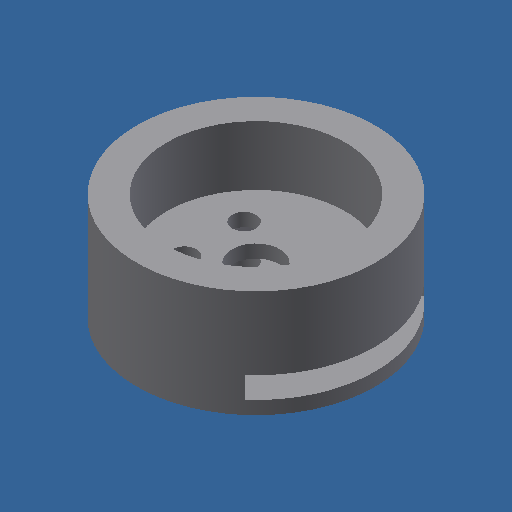
# Autodesk Inventor part: Acople_sensor_hall
Saved by Autodesk Inventor 2025 (Build 290162000, 162)
## iProperties
Created: 2025-09-16
Part Number: Acople_sensor_hall
Material: Generic
Document SubType Name: Modeling
Designer: HP
Density: 1 g/cm^3
Appearance: Default
Author: HP
Autodesk Inventor part; units mm, degrees
ref_plane "XZ Plane" through (0, 0, 0) normal (0, 1, 0) x (-1, 0, 0)
ref_plane "XY Plane" through (0, 0, 0) normal (0, 0, 1) x (1, 0, 0)
sketch "Boceto1" plane through (0, 0, 0) normal (0, 1, 0) x (-1, 0, 0)
  circle A0 centre (0, 0) radius 10
  circle A1 centre (0, 0) radius 7.5
  dimension "d0" = 20
  dimension "d1" = 15
  constraints: 2 centre point, 2 coincident
  measures "d0" diameter of A0
  measures "d1" diameter of A1
extrude "Extrusión1" add sketch "Boceto1" along normal blind 5
sketch "Boceto2" plane through (0, 0, 0) normal (0, -1, 0) x (1, 0, 0)
  circle A0 centre (0, 0) radius 10 projected
extrude "Extrusión2" add sketch "Boceto2" along normal blind 4
ref_plane "Plano de trabajo1" through (10, 0, 0) normal (1, 0, 0) x (0, 1, 0)
sketch "Boceto4" plane through (10, 0, 0) normal (1, 0, 0) x (0, 1, 0)
  line L0 (-4, -10) -> (5, -10) projected
  line L1 (-4, 10) -> (-4, -10) projected
  line L2 (-4, 10) -> (5, 10) projected
  line L3 (5, -10) -> (5, 10) projected
  line L4 (0, 7.5) -> (0, -7.5) projected
  line L5 (-1.1, -7.5) -> (-2.9, -7.5)
  line L6 (-2.9, -7.5) -> (-2.9, 7.5)
  line L7 (-2.9, 7.5) -> (-1.1, 7.5)
  line L8 (-1.1, 7.5) -> (-1.1, -7.5)
  point P0 (0, 0)
  point P1 (-2, -7.5)
  dimension "d7" = 1.8
  dimension "d8" = 15
  dimension "d9" = 2.5
  dimension "d10" = 1.1
  constraints: 8 end point, 2 parallel, 1 horizontal, 1 midpoint, 1 perpendicular
  measures "d7" distance of L6.end L7.end
  measures "d8" distance of L5.end L6.end
  measures "d9" distance from line of point (-2, -7.5) L0
  measures "d10" distance between parallel lines of L8 L4
extrude "Extrusión3" cut sketch "Boceto4" against normal blind 15 contours L5 L6 L7 L8
sketch "Boceto5" plane through (0, 0, 0) normal (0, 1, 0) x (1, 0, 0)
  circle A0 centre (0, 0) radius 7.5 projected
  circle A1 centre (0, 0) radius 7.5 projected
  line L0 (-5, -7.5) -> (-5, 7.5) projected
  circle A2 centre (-3.5, -2.5) radius 1
  circle A3 centre (0, 0) radius 2
  line L1 (0, 0) -> (-5, 0) construction
  circle A4 centre (-3.5, 2.5) radius 1
  dimension "d13" = 2
  dimension "d16" = 4
  dimension "d17" = 1.5
  dimension "d19" = 2.5
  constraints: 3 centre point, 2 end point, 1 coincident, 1 midpoint, 1 symmetric about line, 2 other
  measures "d13" diameter of A2
  measures "d16" diameter of A3
  measures "d17" distance from line of L0 A2.centre
  measures "d19" vertical distance of A2.centre point (0, 0)
extrude "Extrusión4" cut sketch "Boceto5" against normal blind 1.1 contours A3
extrude "Extrusión5" cut sketch "Boceto5" against normal blind 4 contours A2 | A4
